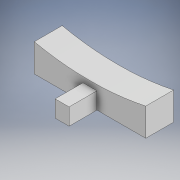
# Autodesk Inventor part: tete_statique
Saved by Autodesk Inventor 2020 (Build 240168000, 168)
## iProperties
Created: 2019-12-28
Part Number: tete_statique
Material: Générique
Document SubType Name: Modeling
Designer: bapti
Density: 1 g/cm^3
Appearance: Par défaut
Author: bapti
Autodesk Inventor part; units mm, degrees
ref_plane "YZ Plane" through (0, 0, 0) normal (1, 0, 0) x (0, 1, 0)
ref_plane "XZ Plane" through (0, 0, 0) normal (0, 1, 0) x (-1, 0, 0)
ref_plane "XY Plane" through (0, 0, 0) normal (0, 0, 1) x (1, 0, 0)
sketch "Esquisse1" plane through (0, 0, 0) normal (0, 0, 1) x (1, 0, 0)
  line L0 (0, 0) -> (0, 10)
  line L1 (0, 0) -> (40, 0)
  line L2 (40, 0) -> (40, 10)
  arc A0 (0, 10) -> (40, 10) centre (20, 103.8936) ccw
  dimension "d0" = 10
  dimension "d1" = 40
  dimension "d3" = 96
  constraints: 6 end point, 2 point on circle, 1 centre point, 1 horizontal, 1 parallel, 1 perpendicular, 1 vertical
  measures "d0" distance of L0.start L0.end
  measures "d1" distance of L0.start L1.end
  measures "d3" radius of A0
extrude "Extrusion1" add sketch "Esquisse1" along normal blind 10
sketch "Esquisse2" plane through (0, 0, 10) normal (0, 0, 1) x (1, 0, 0)
  line L0 (0, 0) -> (40, 0) projected
  line L1 (17.5, 0) -> (22.5, 0)
  line L2 (22.5, 0) -> (22.5, 6)
  line L3 (22.5, 6) -> (17.5, 6)
  line L4 (17.5, 6) -> (17.5, 0)
  line L5 (0, 10) -> (0, 0) projected
  line L6 (0, 7.8936) -> (40, 7.8936) construction
  line L7 (40, 0) -> (40, 10) projected
  arc A0 (0, 10) -> (40, 10) centre (20, 103.8936) ccw projected
  dimension "d6" = 5
  dimension "d8" = 17.5
  dimension "d9" = 40
  dimension "d11" = 6
  constraints: 10 end point, 3 point on line, 2 horizontal, 2 parallel, 1 perpendicular, 1 tangent
  measures "d6" distance of L2.end L3.end
  measures "d8" distance between parallel lines of L4 L5
  measures "d9" distance of L0.start L0.end
  measures "d11" distance of L3.end L1.start
extrude "Extrusion2" add sketch "Esquisse2" along normal blind 10 contours L4 L3 L2 L0
equation "\"d8\" = 0.5 * d9 - 0.5 * d6"
